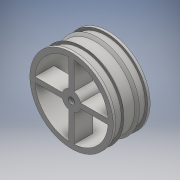
# Autodesk Inventor part: OSV Specific Wheel #2
Saved by Autodesk Inventor 2016 (Build 200138000, 138)
## iProperties
Created: 2016-04-05
Part Number: OSV Specific Wheel #2
Material: Generic
Document SubType Name: Modeling
Designer: Kenneth Daniel
Density: 1 g/cm^3
Appearance: Default
Author: Kenneth Daniel
Autodesk Inventor part; units mm, degrees
ref_plane "YZ Plane" through (0, 0, 0) normal (1, 0, 0) x (0, 1, 0)
ref_plane "XZ Plane" through (0, 0, 0) normal (0, 1, 0) x (-1, 0, 0)
ref_plane "XY Plane" through (0, 0, 0) normal (0, 0, 1) x (1, 0, 0)
sketch "Sketch1" plane through (0, 0, 0) normal (0, 0, 1) x (1, 0, 0)
  line L0 (0, 0) -> (31.095, 0)
  line L1 (31.095, 0) -> (31.095, 14.685)
  line L2 (31.095, 14.685) -> (33.095, 14.685)
  line L3 (33.095, 14.685) -> (33.095, 12.685)
  line L4 (33.095, 12.685) -> (31.095, 12.685)
  line L5 (31.095, 0) -> (31.095, 6.28)
  line L6 (31.095, 6.28) -> (33.095, 6.28)
  line L7 (33.095, 6.28) -> (31.095, 4.3618)
  line L8 (31.095, -14.685) -> (33.095, -14.685)
  line L9 (33.095, -14.685) -> (33.095, -12.685)
  line L10 (33.095, -12.685) -> (31.095, -12.685)
  line L11 (31.095, -6.28) -> (33.095, -6.28)
  line L12 (33.095, -6.28) -> (31.095, -4.3618)
  line L13 (31.095, 14.685) -> (29.095, 14.685)
  line L14 (29.095, 14.685) -> (29.095, -14.685)
  line L15 (29.095, -14.685) -> (31.095, -14.685)
  line L16 (33.095, -6.28) -> (31.095, -4.3618)
  line L17 (31.095, 0) -> (31.095, -4.3618)
  line L18 (31.095, -6.28) -> (31.095, -14.685)
  line L19 (0, -20.559) -> (0, 20.559) projected
  dimension "d0" = 31.095
  dimension "d1" = 14.685
  dimension "d2" = 2
  dimension "d3" = 2
  dimension "d4" = 6.28
  dimension "d5" = 2
  dimension "d6" = 2
  constraints: 38 end point, 7 symmetric about line, 6 perpendicular, 6 point on line, 2 horizontal, 1 collinear
  measures "d0" distance of L0.start L0.end
  measures "d1" distance of L0.end L1.end
  measures "d2" distance of L1.end L2.end
  measures "d3" distance of L2.end L3.end
  measures "d4" distance of L0.end L5.end
  measures "d5" distance of L5.end L6.end
  measures "d6" distance of L1.end L13.end
revolve "Revolution1" add sketch "Sketch1" angle 360 about axis through (0, -10, 0) along (0, 1, 0)
sketch "Sketch2" plane through (0, -14.685, 0) normal (0, -1, 0) x (1, 0, 0)
  circle A0 centre (0, 0) radius 29.095
  line L0 (0, 0) -> (-2, 0)
  line L1 (-2, 0) -> (2, 0)
  line L2 (-2, 0) -> (2, 0)
  line L3 (2, 0) -> (2, 29.0262)
  line L4 (-2, 29.0262) -> (-2, 0)
  circle A1 centre (0, 0) radius 7.5
  dimension "d8" = 2
  dimension "d9" = 4
  dimension "d10" = 15
  constraints: 10 end point, 2 centre point, 2 coincident, 2 horizontal, 2 point on circle, 1 parallel, 1 perpendicular, 1 point on line
  measures "d8" distance of L0.start L0.end
  measures "d9" distance of L0.end L1.end
  measures "d10" diameter of A1
extrude "Extrusion1" add sketch "Sketch2" against normal blind 15 contours L3 A1 L4 A0 | A1 L4 L0 L1 L3 | L3 L1 L0 L4 A1 picked at (-0.2224, 14.6756)
pattern_circular "Circular Pattern1" count 4 over 360 about axis through (0, -14.685, 0) along (0, 1, 0) of "Extrusion1"
sketch "Sketch3" plane through (0, -14.685, 0) normal (0, -1, 0) x (1, 0, 0)
  circle A0 centre (0, 0) radius 2.5
  dimension "d16" = 5
  constraints: 1 centre point, 1 coincident
  measures "d16" diameter of A0
extrude "Extrusion2" cut sketch "Sketch3" against normal blind 15
body "Solid1"
